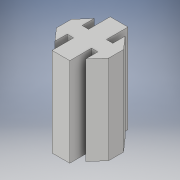
# Autodesk Inventor part: 20X20 lift conecter
Saved by Autodesk Inventor 2019 (Build 230136000, 136)
## iProperties
Created: 2018-10-23
Part Number: 20X20 lift conecter
Material: Generic
Document SubType Name: Modeling
Designer: User
Density: 1 g/cm^3
Appearance: Default
Author: User
Autodesk Inventor part; units mm, degrees
ref_plane "YZ Plane" through (0, 0, 0) normal (1, 0, 0) x (0, 1, 0)
ref_plane "XZ Plane" through (0, 0, 0) normal (0, 1, 0) x (-1, 0, 0)
ref_plane "XY Plane" through (0, 0, 0) normal (0, 0, 1) x (1, 0, 0)
sketch "Sketch1" plane through (0, 0, 0) normal (0, 1, 0) x (-1, 0, 0)
  line L0 (0, 0) -> (5.08, 0)
  line L1 (5.08, 0) -> (5.08, -16.637)
  line L2 (5.08, -16.637) -> (0, -16.637)
  line L3 (0, -16.637) -> (0, 0)
  line L4 (-1.8542, -6.1892) -> (6.9342, -6.1892)
  line L5 (6.9342, -6.1892) -> (6.9342, -10.4478)
  line L6 (6.9342, -10.4478) -> (-1.8542, -10.4478)
  line L7 (-1.8542, -10.4478) -> (-1.8542, -6.1892)
  line L8 (10.0076, -6.1892) -> (10.0076, -10.4478)
  line L9 (6.9342, -13.9319) -> (6.9342, -2.7051)
  line L10 (-4.9276, -6.1892) -> (-4.9276, -10.4478)
  line L11 (-1.8542, -13.9319) -> (-1.8542, -2.7051)
  line L12 (6.9342, -13.9319) -> (10.0076, -10.4478)
  line L13 (6.9342, -2.7051) -> (10.0076, -6.1892)
  line L14 (-1.8542, -2.7051) -> (-4.9276, -6.1892)
  line L15 (-1.8542, -13.9319) -> (-4.9276, -10.4478)
  dimension "d0" = 5.08
  dimension "d1" = 16.637
  dimension "d2" = 1.8542
  dimension "d3" = 1.8542
  dimension "d4" = 4.2585
  dimension "d6" = 6.1893
  dimension "d9" = 3.0734
  dimension "d11" = 0
  dimension "d12" = 0
  dimension "d15" = 11.2268
  dimension "d16" = 11.2268
  dimension "d17" = 2.7051
  dimension "d18" = 2.7051
  dimension "d19" = 3.0734
  constraints: 32 end point, 7 parallel, 2 horizontal, 2 perpendicular, 1 point on line
  measures "d0" distance of L1.end L2.end
  measures "d1" distance of L0.end L1.end
  measures "d2" distance between parallel lines of L5 L1
  measures "d3" distance between parallel lines of L7 L3
  measures "d4" distance of L6.end L4.start
  measures "d6" distance between parallel lines of L6 L2
  measures "d9" distance between parallel lines of L8 L9
  measures "d11" distance between parallel lines of L7 L11
  measures "d12" distance between parallel lines of L5 L9
  measures "d15" distance of L11.end L11.start
  measures "d16" distance of L9.start L9.end
  measures "d17" distance from line of L2 L9.start
  measures "d18" distance from line of L2 L11.start
  measures "d19" distance between parallel lines of L7 L10
extrude "Extrusion1" add sketch "Sketch1" along normal blind 25.4
equation "\"d3\" = d2"
equation "\"d6\" = -0.5 * d4 + 0.5 * d1"
equation "\"d16\" = d15"
equation "\"d17\" = -0.5 * d16 + 0.5 * d1"
equation "\"d18\" = d17"
equation "\"d19\" = d9"
body "Solid1"
